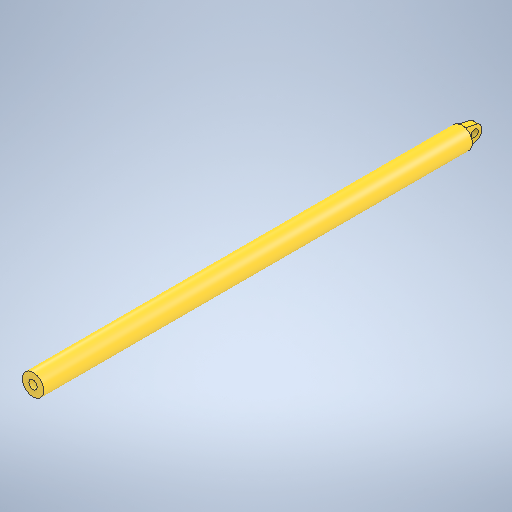
# Autodesk Inventor part: Parth_Cylinder2
Saved by Autodesk Inventor 2025 (Build 290162000, 162)
## iProperties
Created: 2024-11-03
Part Number: Parth_Cylinder2
Material: Generic
Document SubType Name: Modeling
Designer: kalep
Density: 1 g/cm^3
Appearance: Default
Author: kalep
Autodesk Inventor part; units mm, degrees
ref_plane "YZ Plane" through (0, 0, 0) normal (1, 0, 0) x (0, 1, 0)
ref_plane "XZ Plane" through (0, 0, 0) normal (0, 1, 0) x (-1, 0, 0)
ref_plane "XY Plane" through (0, 0, 0) normal (0, 0, 1) x (1, 0, 0)
sketch "Sketch1" plane through (0, 0, 0) normal (0, 0, 1) x (1, 0, 0)
  circle A0 centre (0, 0) radius 50
  dimension "d0" = 100
  constraints: 1 centre point, 1 coincident
  measures "d0" diameter of A0
extrude "Extrusion1" add sketch "Sketch1" along normal blind 2000
sketch "Sketch2" plane through (0, 0, 0) normal (1, 0, 0) x (0, 1, 0)
  line L0 (50, 0) -> (-50, 0) projected
  arc A0 (-31.5648, -59.3002) -> (32.3259, -59.3002) centre (0.3805, -45) ccw
  line L1 (32.3259, -59.3002) -> (45.3805, 0)
  circle A1 centre (0.3805, -45) radius 17.5
  line L2 (-45, 0) -> (-31.5648, -59.3002)
  point P0 (0, 0)
  point P1 (0, 0)
  dimension "d3" = 35
  dimension "d4" = 35
  dimension "d5" = 45
  dimension "d6" = 45
  dimension "d7" = 45
  constraints: 4 end point, 2 centre point, 2 point on circle, 2 point on line, 1 concentric, 1 midpoint
  measures "d3" radius of A0
  measures "d4" diameter of A1
  measures "d5" distance from line of L0 A0.centre
  measures "d6" horizontal distance of A1.centre L1.end
  measures "d7" distance of point (0, 0) L2.start
extrude "Extrusion2" add sketch "Sketch2" along normal mid plane 30
shell "Shell1" thickness 30 removed faces 1 at (9.39, -8.8667, 2000)
body "Solid1"
